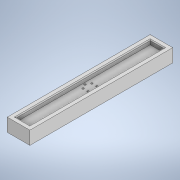
# Autodesk Inventor part: enclosure_btm
Saved by Autodesk Inventor 2020 (Build 240168000, 168)
## iProperties
Created: 2020-04-01
Part Number: enclosure_btm
Material: Generic
Document SubType Name: Modeling
Designer: Clevo
Density: 1 g/cm^3
Appearance: Default
Author: Clevo
Autodesk Inventor part; units mm, degrees
ref_plane "YZ Plane" through (0, 0, 0) normal (1, 0, 0) x (0, 1, 0)
ref_plane "XZ Plane" through (0, 0, 0) normal (0, 1, 0) x (-1, 0, 0)
ref_plane "XY Plane" through (0, 0, 0) normal (0, 0, 1) x (1, 0, 0)
sketch "Sketch1" plane through (0, 0, 0) normal (0, 1, 0) x (-1, 0, 0)
  line L0 (-15.7, -152.5) -> (15.7, -152.5)
  line L1 (15.7, -152.5) -> (15.7, 152.5)
  line L2 (15.7, 152.5) -> (-15.7, 152.5)
  line L3 (-15.7, 152.5) -> (-15.7, -152.5)
  line L4 (-15.7, -152.5) -> (15.7, 152.5) construction
  line L5 (15.7, -152.5) -> (-15.7, 152.5) construction
  line L6 (25.7, 162.5) -> (25.7, -162.5)
  line L7 (25.7, -162.5) -> (-25.7, -162.5)
  line L8 (-25.7, -162.5) -> (-25.7, 162.5)
  line L9 (-25.7, 162.5) -> (25.7, 162.5)
  point P0 (0, 0)
  dimension "d0" = 31.4
  dimension "d1" = 305
  dimension "d2" = 10
  constraints: 20 end point, 4 parallel, 2 midpoint, 2 perpendicular, 1 horizontal, 3 other
  measures "d0" distance of L1.end L2.end
  measures "d1" distance of L0.end L1.end
  measures "d2" distance between parallel lines of L1 L6
extrude "Extrusion1" add sketch "Sketch1" along normal blind 10
sketch "Sketch2" plane through (0, 0, 0) normal (0, -1, 0) x (1, 0, 0)
  line L0 (25.7, 162.5) -> (25.7, -162.5) projected
  line L1 (-25.7, 162.5) -> (25.7, 162.5) projected
  line L2 (-25.7, -162.5) -> (-25.7, 162.5) projected
  line L3 (25.7, -162.5) -> (-25.7, -162.5) projected
  line L4 (-15.7, 152.5) -> (-15.7, -152.5) projected
  line L5 (15.7, 152.5) -> (-15.7, 152.5) projected
  line L6 (15.7, -152.5) -> (15.7, 152.5) projected
  line L7 (-15.7, -152.5) -> (15.7, -152.5) projected
  point P0 (0, 0)
extrude "Extrusion2" add sketch "Sketch2" along normal blind 20 contours L0 L3 L2 L1 | L5 L6 L7 L4
sketch "Sketch4" plane through (0, -20, 0) normal (0, -1, 0) x (1, 0, 0)
  point P0 (0, 0)
  point P1 (11.5, 0)
  dimension "d14" = 11.5
  constraints: 1 horizontal alignment
  measures "d14" distance of point (0, 0) point (11.5, 0)
hole "Hole2" at (11.5, -20, 0) direction (0, 1, 0) diameter 4.134 end through all thread size "M5x0.8" class "6H" standard "ANSI Metric M Profile"
pattern_circular "Circular Pattern1" count 6 over 360 about axis through (0, -10, 0) along (0, 1, 0) of "Hole2"
fillet "Fillet1" radius 2 4 edges at (-15.7, 10, 0) (0, 10, -152.5) (15.7, 10, 0) (0, 10, 152.5)
body "Solid1"
